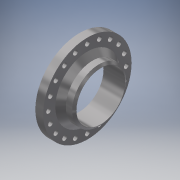
# Autodesk Inventor part: Weldneck Flange 14 in
Saved by Autodesk Inventor 2016 (Build 200138000, 138)
## iProperties
Created: 2018-11-05
Part Number: Weldneck Flange 14 in
Material: ASTM A105 Gr.B
Document SubType Name: Modeling
Designer: Wijaya
Mass: 88692 g
Surface Area: 7601.79 cm^2
Volume: 11298.3 cm^3
Density: 7.85 g/cm^3
Appearance: Semi-Polished
Author: Wijaya
Autodesk Inventor part; units mm, degrees
note: some values were not read from the file. Chosen so that the rebuilt part matches the saved one: direction of "Hole1".
ref_plane "YZ Plane" through (0, 0, 0) normal (1, 0, 0) x (0, 1, 0)
ref_plane "XZ Plane" through (0, 0, 0) normal (0, 1, 0) x (-1, 0, 0)
ref_plane "XY Plane" through (0, 0, 0) normal (0, 0, 1) x (1, 0, 0)
sketch "Sketch1" plane through (0, 0, 0) normal (0, 0, 1) x (1, 0, 0)
  line L0 (0, 0) -> (-156.093, 0)
  line L1 (0, 162.7083) -> (0, 161.1083)
  line L2 (0, 162.7083) -> (-11.5803, 177.8)
  line L3 (-11.5803, 177.8) -> (-53.9, 177.8)
  line L4 (-53.9, 177.8) -> (-88.6, 212.5)
  line L5 (-88.6, 212.5) -> (-88.6, 292.5)
  line L6 (-88.6, 292.5) -> (-141, 292.5)
  line L7 (-141, 292.5) -> (-141, 212.5)
  line L8 (-141, 212.5) -> (-143, 212.5)
  line L9 (-143, 212.5) -> (-143, 161.1083)
  line L10 (-143, 161.1083) -> (0, 161.1083)
  dimension "d0" = 37.5
  dimension "d2" = 2
  dimension "d3" = 52.4
  dimension "d4" = 585
  dimension "d5" = 322.2165
  dimension "d7" = 425
  dimension "d8" = 1.6
  dimension "d9" = 425
  dimension "d10" = 45
  dimension "d11" = 355.6
  dimension "d24" = 141
  constraints: 22 end point, 4 perpendicular, 3 horizontal, 2 vertical, 1 vertical alignment
  measures "d0" angle of L1 L2
  measures "d2" distance of L7.end L8.end
  measures "d3" distance of L5.end L6.end
  measures "d4" diameter of L6 L0
  measures "d5" diameter of L10 L0
  measures "d7" diameter of L8 L0
  measures "d8" distance of L1.start L1.end
  measures "d9" diameter of L4.end L0
  measures "d10" angle of L5 L4
  measures "d11" diameter of L3 L0
  measures "d24" distance between parallel lines of L1 L7
revolve "Revolution1" add sketch "Sketch1" angle 360 about axis through (0, 0, 0) along (-1, 0, 0)
sketch "Sketch2" plane through (-88.6, 0, 0) normal (1, 0, 0) x (0, 0, -1)
  point P0 (0, 0)
  point P1 (0, 257.2)
  dimension "d13" = 257.2
  constraints: 1 vertical alignment
  measures "d13" distance of point (0, 0) point (0, 257.2)
hole "Hole1" at (-88.6, 257.2, 0) direction (-1, 0, 0) diameter 31.75 end up to surface
pattern_circular "Circular Pattern1" count 20 over 360 about axis through (-71.5, 0, 0) along (1, 0, 0) of "Hole1"
body "Solid1"
